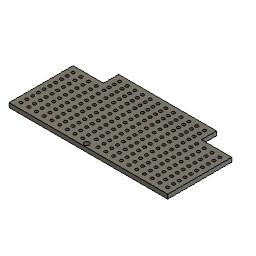
bottom mounting plate (Autodesk Fusion 360 design; units mm, degrees)
Autodesk Fusion 360 part; units mm, degrees
sketch "Sketch1" plane through (0, 0, 0) normal (0, 1, 0) x (1, 0, 0)
  line L0 (235, 95) -> (190, 95)
  line L1 (190, 95) -> (190, 117.5)
  line L2 (45, 117.5) -> (45, 95)
  line L3 (45, 95) -> (0, 95)
  line L4 (0, 0) -> (0, 95)
  line L5 (45, 117.5) -> (190, 117.5)
  line L6 (235, 95) -> (235, 0)
  line L7 (0, 0) -> (235, 0)
  circle A0 centre (110, 5) radius 3.75
  circle A1 centre (9, 9) radius 2.25
  circle A2 centre (20.4211, 9) radius 2.25
  circle A3 centre (31.8421, 9) radius 2.25
  circle A4 centre (43.2632, 9) radius 2.25
  circle A5 centre (54.6842, 9) radius 2.25
  circle A6 centre (66.1053, 9) radius 2.25
  circle A7 centre (77.5263, 9) radius 2.25
  circle A8 centre (88.9474, 9) radius 2.25
  circle A9 centre (100.3684, 9) radius 2.25
  circle A10 centre (123.2105, 9) radius 2.25
  circle A11 centre (134.6316, 9) radius 2.25
  circle A12 centre (146.0526, 9) radius 2.25
  circle A13 centre (157.4737, 9) radius 2.25
  circle A14 centre (168.8947, 9) radius 2.25
  circle A15 centre (180.3158, 9) radius 2.25
  circle A16 centre (191.7368, 9) radius 2.25
  circle A17 centre (203.1579, 9) radius 2.25
  circle A18 centre (214.5789, 9) radius 2.25
  circle A19 centre (226, 9) radius 2.25
  circle A20 centre (9, 17.5551) radius 2.25
  circle A21 centre (20.4211, 17.5551) radius 2.25
  circle A22 centre (31.8421, 17.5551) radius 2.25
  circle A23 centre (43.2632, 17.5551) radius 2.25
  circle A24 centre (54.6842, 17.5551) radius 2.25
  circle A25 centre (66.1053, 17.5551) radius 2.25
  circle A26 centre (77.5263, 17.5551) radius 2.25
  circle A27 centre (88.9474, 17.5551) radius 2.25
  circle A28 centre (100.3684, 17.5551) radius 2.25
  circle A29 centre (111.7895, 17.5551) radius 2.25
  circle A30 centre (123.2105, 17.5551) radius 2.25
  circle A31 centre (134.6316, 17.5551) radius 2.25
  circle A32 centre (146.0526, 17.5551) radius 2.25
  circle A33 centre (157.4737, 17.5551) radius 2.25
  circle A34 centre (168.8947, 17.5551) radius 2.25
  circle A35 centre (180.3158, 17.5551) radius 2.25
  circle A36 centre (191.7368, 17.5551) radius 2.25
  circle A37 centre (203.1579, 17.5551) radius 2.25
  circle A38 centre (214.5789, 17.5551) radius 2.25
  circle A39 centre (226, 17.5551) radius 2.25
  circle A40 centre (9, 26.1102) radius 2.25
  circle A41 centre (20.4211, 26.1102) radius 2.25
  circle A42 centre (31.8421, 26.1102) radius 2.25
  circle A43 centre (43.2632, 26.1102) radius 2.25
  circle A44 centre (54.6842, 26.1102) radius 2.25
  circle A45 centre (66.1053, 26.1102) radius 2.25
  circle A46 centre (77.5263, 26.1102) radius 2.25
  circle A47 centre (88.9474, 26.1102) radius 2.25
  circle A48 centre (100.3684, 26.1102) radius 2.25
  circle A49 centre (111.7895, 26.1102) radius 2.25
  circle A50 centre (123.2105, 26.1102) radius 2.25
  circle A51 centre (134.6316, 26.1102) radius 2.25
  circle A52 centre (146.0526, 26.1102) radius 2.25
  circle A53 centre (157.4737, 26.1102) radius 2.25
  circle A54 centre (168.8947, 26.1102) radius 2.25
  circle A55 centre (180.3158, 26.1102) radius 2.25
  circle A56 centre (191.7368, 26.1102) radius 2.25
  circle A57 centre (203.1579, 26.1102) radius 2.25
  circle A58 centre (214.5789, 26.1102) radius 2.25
  circle A59 centre (226, 26.1102) radius 2.25
  circle A60 centre (9, 34.6653) radius 2.25
  circle A61 centre (20.4211, 34.6653) radius 2.25
  circle A62 centre (31.8421, 34.6653) radius 2.25
  circle A63 centre (43.2632, 34.6653) radius 2.25
  circle A64 centre (54.6842, 34.6653) radius 2.25
  circle A65 centre (66.1053, 34.6653) radius 2.25
  circle A66 centre (77.5263, 34.6653) radius 2.25
  circle A67 centre (88.9474, 34.6653) radius 2.25
  circle A68 centre (100.3684, 34.6653) radius 2.25
  circle A69 centre (111.7895, 34.6653) radius 2.25
  circle A70 centre (123.2105, 34.6653) radius 2.25
  circle A71 centre (134.6316, 34.6653) radius 2.25
  circle A72 centre (146.0526, 34.6653) radius 2.25
  circle A73 centre (157.4737, 34.6653) radius 2.25
  circle A74 centre (168.8947, 34.6653) radius 2.25
  circle A75 centre (180.3158, 34.6653) radius 2.25
  circle A76 centre (191.7368, 34.6653) radius 2.25
  circle A77 centre (203.1579, 34.6653) radius 2.25
  circle A78 centre (214.5789, 34.6653) radius 2.25
  circle A79 centre (226, 34.6653) radius 2.25
  circle A80 centre (9, 43.2204) radius 2.25
  circle A81 centre (20.4211, 43.2204) radius 2.25
  circle A82 centre (31.8421, 43.2204) radius 2.25
  circle A83 centre (43.2632, 43.2204) radius 2.25
  circle A84 centre (54.6842, 43.2204) radius 2.25
  circle A85 centre (66.1053, 43.2204) radius 2.25
  circle A86 centre (77.5263, 43.2204) radius 2.25
  circle A87 centre (88.9474, 43.2204) radius 2.25
  circle A88 centre (100.3684, 43.2204) radius 2.25
  circle A89 centre (111.7895, 43.2204) radius 2.25
  circle A90 centre (123.2105, 43.2204) radius 2.25
  circle A91 centre (134.6316, 43.2204) radius 2.25
  circle A92 centre (146.0526, 43.2204) radius 2.25
  circle A93 centre (157.4737, 43.2204) radius 2.25
  circle A94 centre (168.8947, 43.2204) radius 2.25
  circle A95 centre (180.3158, 43.2204) radius 2.25
  circle A96 centre (191.7368, 43.2204) radius 2.25
  circle A97 centre (203.1579, 43.2204) radius 2.25
  circle A98 centre (214.5789, 43.2204) radius 2.25
  circle A99 centre (226, 43.2204) radius 2.25
  circle A100 centre (9, 51.7756) radius 2.25
  circle A101 centre (20.4211, 51.7756) radius 2.25
  circle A102 centre (31.8421, 51.7756) radius 2.25
  circle A103 centre (43.2632, 51.7756) radius 2.25
  circle A104 centre (54.6842, 51.7756) radius 2.25
  circle A105 centre (66.1053, 51.7756) radius 2.25
  circle A106 centre (77.5263, 51.7756) radius 2.25
  circle A107 centre (88.9474, 51.7756) radius 2.25
  circle A108 centre (100.3684, 51.7756) radius 2.25
  circle A109 centre (111.7895, 51.7756) radius 2.25
  circle A110 centre (123.2105, 51.7756) radius 2.25
  circle A111 centre (134.6316, 51.7756) radius 2.25
  circle A112 centre (146.0526, 51.7756) radius 2.25
  circle A113 centre (157.4737, 51.7756) radius 2.25
  circle A114 centre (168.8947, 51.7756) radius 2.25
  circle A115 centre (180.3158, 51.7756) radius 2.25
  circle A116 centre (191.7368, 51.7756) radius 2.25
  circle A117 centre (203.1579, 51.7756) radius 2.25
  circle A118 centre (214.5789, 51.7756) radius 2.25
  circle A119 centre (226, 51.7756) radius 2.25
  circle A120 centre (9, 60.3307) radius 2.25
  circle A121 centre (20.4211, 60.3307) radius 2.25
  circle A122 centre (31.8421, 60.3307) radius 2.25
  circle A123 centre (43.2632, 60.3307) radius 2.25
  circle A124 centre (54.6842, 60.3307) radius 2.25
  circle A125 centre (66.1053, 60.3307) radius 2.25
  circle A126 centre (77.5263, 60.3307) radius 2.25
  circle A127 centre (88.9474, 60.3307) radius 2.25
  circle A128 centre (100.3684, 60.3307) radius 2.25
  circle A129 centre (111.7895, 60.3307) radius 2.25
  circle A130 centre (123.2105, 60.3307) radius 2.25
  circle A131 centre (134.6316, 60.3307) radius 2.25
  circle A132 centre (146.0526, 60.3307) radius 2.25
  circle A133 centre (157.4737, 60.3307) radius 2.25
  circle A134 centre (168.8947, 60.3307) radius 2.25
  circle A135 centre (180.3158, 60.3307) radius 2.25
  circle A136 centre (191.7368, 60.3307) radius 2.25
  circle A137 centre (203.1579, 60.3307) radius 2.25
  circle A138 centre (214.5789, 60.3307) radius 2.25
  circle A139 centre (226, 60.3307) radius 2.25
  circle A140 centre (9, 68.8858) radius 2.25
  circle A141 centre (20.4211, 68.8858) radius 2.25
  circle A142 centre (31.8421, 68.8858) radius 2.25
  circle A143 centre (43.2632, 68.8858) radius 2.25
  circle A144 centre (54.6842, 68.8858) radius 2.25
  circle A145 centre (66.1053, 68.8858) radius 2.25
  circle A146 centre (77.5263, 68.8858) radius 2.25
  circle A147 centre (88.9474, 68.8858) radius 2.25
  circle A148 centre (100.3684, 68.8858) radius 2.25
  circle A149 centre (111.7895, 68.8858) radius 2.25
  circle A150 centre (123.2105, 68.8858) radius 2.25
  circle A151 centre (134.6316, 68.8858) radius 2.25
  circle A152 centre (146.0526, 68.8858) radius 2.25
  circle A153 centre (157.4737, 68.8858) radius 2.25
  circle A154 centre (168.8947, 68.8858) radius 2.25
  circle A155 centre (180.3158, 68.8858) radius 2.25
  circle A156 centre (191.7368, 68.8858) radius 2.25
  circle A157 centre (203.1579, 68.8858) radius 2.25
  circle A158 centre (214.5789, 68.8858) radius 2.25
  circle A159 centre (226, 68.8858) radius 2.25
  circle A160 centre (9, 77.4409) radius 2.25
  circle A161 centre (20.4211, 77.4409) radius 2.25
  circle A162 centre (31.8421, 77.4409) radius 2.25
  circle A163 centre (43.2632, 77.4409) radius 2.25
  circle A164 centre (54.6842, 77.4409) radius 2.25
  circle A165 centre (66.1053, 77.4409) radius 2.25
  circle A166 centre (77.5263, 77.4409) radius 2.25
  circle A167 centre (88.9474, 77.4409) radius 2.25
  circle A168 centre (100.3684, 77.4409) radius 2.25
  circle A169 centre (111.7895, 77.4409) radius 2.25
  circle A170 centre (123.2105, 77.4409) radius 2.25
  circle A171 centre (134.6316, 77.4409) radius 2.25
  circle A172 centre (146.0526, 77.4409) radius 2.25
  circle A173 centre (157.4737, 77.4409) radius 2.25
  circle A174 centre (168.8947, 77.4409) radius 2.25
  circle A175 centre (180.3158, 77.4409) radius 2.25
  circle A176 centre (191.7368, 77.4409) radius 2.25
  circle A177 centre (203.1579, 77.4409) radius 2.25
  circle A178 centre (214.5789, 77.4409) radius 2.25
  circle A179 centre (226, 77.4409) radius 2.25
  circle A180 centre (9, 85.996) radius 2.25
  circle A181 centre (20.4211, 85.996) radius 2.25
  circle A182 centre (31.8421, 85.996) radius 2.25
  circle A183 centre (43.2632, 85.996) radius 2.25
  circle A184 centre (54.6842, 85.996) radius 2.25
  circle A185 centre (66.1053, 85.996) radius 2.25
  circle A186 centre (77.5263, 85.996) radius 2.25
  circle A187 centre (88.9474, 85.996) radius 2.25
  circle A188 centre (100.3684, 85.996) radius 2.25
  circle A189 centre (111.7895, 85.996) radius 2.25
  circle A190 centre (123.2105, 85.996) radius 2.25
  circle A191 centre (134.6316, 85.996) radius 2.25
  circle A192 centre (146.0526, 85.996) radius 2.25
  circle A193 centre (157.4737, 85.996) radius 2.25
  circle A194 centre (168.8947, 85.996) radius 2.25
  circle A195 centre (180.3158, 85.996) radius 2.25
  circle A196 centre (191.7368, 85.996) radius 2.25
  circle A197 centre (203.1579, 85.996) radius 2.25
  circle A198 centre (214.5789, 85.996) radius 2.25
  circle A199 centre (226, 85.996) radius 2.25
  circle A200 centre (66.1142, 85.996) radius 2.25
  circle A201 centre (77.5442, 85.996) radius 2.25
  circle A202 centre (88.9742, 85.996) radius 2.25
  circle A203 centre (100.4042, 85.996) radius 2.25
  circle A204 centre (111.8342, 85.996) radius 2.25
  circle A205 centre (123.2642, 85.996) radius 2.25
  circle A206 centre (134.6942, 85.996) radius 2.25
  circle A207 centre (146.1242, 85.996) radius 2.25
  circle A208 centre (157.5542, 85.996) radius 2.25
  circle A209 centre (168.9842, 85.996) radius 2.25
  circle A210 centre (180.4142, 85.996) radius 2.25
  circle A211 centre (191.8442, 85.996) radius 2.25
  circle A212 centre (54.6842, 93.616) radius 2.25
  circle A213 centre (66.1142, 93.616) radius 2.25
  circle A214 centre (77.5442, 93.616) radius 2.25
  circle A215 centre (88.9742, 93.616) radius 2.25
  circle A216 centre (100.4042, 93.616) radius 2.25
  circle A217 centre (111.8342, 93.616) radius 2.25
  circle A218 centre (123.2642, 93.616) radius 2.25
  circle A219 centre (134.6942, 93.616) radius 2.25
  circle A220 centre (146.1242, 93.616) radius 2.25
  circle A221 centre (157.5542, 93.616) radius 2.25
  circle A222 centre (168.9842, 93.616) radius 2.25
  circle A223 centre (180.4142, 93.616) radius 2.25
  circle A224 centre (54.6842, 101.236) radius 2.25
  circle A225 centre (66.1142, 101.236) radius 2.25
  circle A226 centre (77.5442, 101.236) radius 2.25
  circle A227 centre (88.9742, 101.236) radius 2.25
  circle A228 centre (100.4042, 101.236) radius 2.25
  circle A229 centre (111.8342, 101.236) radius 2.25
  circle A230 centre (123.2642, 101.236) radius 2.25
  circle A231 centre (134.6942, 101.236) radius 2.25
  circle A232 centre (146.1242, 101.236) radius 2.25
  circle A233 centre (157.5542, 101.236) radius 2.25
  circle A234 centre (168.9842, 101.236) radius 2.25
  circle A235 centre (180.4142, 101.236) radius 2.25
  circle A236 centre (54.6842, 108.856) radius 2.25
  circle A237 centre (66.1142, 108.856) radius 2.25
  circle A238 centre (77.5442, 108.856) radius 2.25
  circle A239 centre (88.9742, 108.856) radius 2.25
  circle A240 centre (100.4042, 108.856) radius 2.25
  circle A241 centre (111.8342, 108.856) radius 2.25
  circle A242 centre (123.2642, 108.856) radius 2.25
  circle A243 centre (134.6942, 108.856) radius 2.25
  circle A244 centre (146.1242, 108.856) radius 2.25
  circle A245 centre (157.5542, 108.856) radius 2.25
  circle A246 centre (168.9842, 108.856) radius 2.25
  circle A247 centre (180.4142, 108.856) radius 2.25
  dimension "d10" = 45
  dimension "d11" = 22.5
  dimension "d12" = 45
  dimension "d16" = 95
  dimension "d18" = 95
  dimension "d23" = 7.5
  dimension "d26" = 4.5
  dimension "d30" = 217
  dimension "d31" = 76.996
  dimension "d34" = 137.16
  dimension "d35" = 22.86
  constraint coincident L4.start L7.start
  constraint perpendicular L3 L4
  constraint perpendicular L1 L5
  constraint perpendicular L6 L7
  measures "d10" distance of L0.start L0.end
  measures "d11" distance of L2.start L2.end
  measures "d12" distance of L2.end L3.end
  measures "d16" distance of L4.start L3.end
  measures "d18" distance of L6.end L0.start
  measures "d23" diameter of A0
  measures "d26" diameter of A1
extrude "Extrude1" add sketch "Sketch1" along normal blind 6.35
